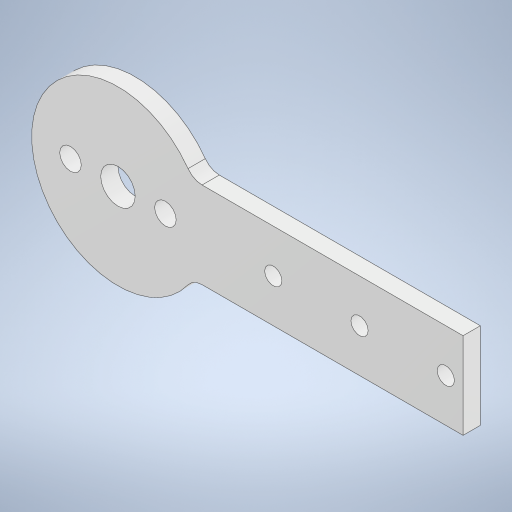
# Autodesk Inventor part: cutter_board
Saved by Autodesk Inventor 2024 (Build 280153000, 153)
## iProperties
Created: 2025-03-05
Part Number: cutter_board
Material: ABS プラスチック
Document SubType Name: Modeling
Designer: 1412z
Density: 1.06 g/cm^3
Appearance: 滑らか - 白
Author: 1412z
Autodesk Inventor part; units mm, degrees
ref_plane "YZ Plane" through (0, 0, 0) normal (1, 0, 0) x (0, 1, 0)
ref_plane "XZ Plane" through (0, 0, 0) normal (0, 1, 0) x (-1, 0, 0)
ref_plane "XY Plane" through (0, 0, 0) normal (0, 0, 1) x (1, 0, 0)
sketch "スケッチ5" plane through (0, 0, 0) normal (0, 0, 1) x (1, 0, 0)
  circle A0 centre (0, 0) radius 2
  circle A1 centre (0, 0) radius 10
  line L0 (0, 0) -> (40, 0)
  line L1 (40, 0) -> (40, -5)
  line L2 (40, -5) -> (8.6603, -5)
  line L3 (40, 0) -> (40, 5)
  line L4 (40, 5) -> (8.6603, 5)
  circle A2 centre (18, 0) radius 1
  circle A3 centre (28, 0) radius 1
  circle A4 centre (38, 0) radius 1
  circle A5 centre (0, 0) radius 5.5
  circle A6 centre (-5.5, 0) radius 1.25
  circle A7 centre (5.5, 0) radius 1.25
  dimension "d31" = 4
  dimension "d32" = 20
  dimension "d33" = 40
  dimension "d34" = 5
  dimension "d35" = 5
  dimension "d36" = 2
  dimension "d37" = 2
  dimension "d38" = 2
  dimension "d39" = 11
  dimension "d40" = 2.5
  dimension "d41" = 2.5
  constraints: 10 end point, 8 centre point, 5 point on line, 4 point on circle, 3 coincident, 3 perpendicular, 1 horizontal
  measures "d31" diameter of A0
  measures "d32" diameter of A1
  measures "d33" distance of L0.start L0.end
  measures "d34" distance of L0.end L1.end
  measures "d35" distance of L0.end L3.end
  measures "d36" diameter of A2
  measures "d37" diameter of A3
  measures "d38" diameter of A4
  measures "d39" diameter of A5
  measures "d40" diameter of A6
  measures "d41" diameter of A7
extrude "押し出し5" add sketch "スケッチ5" along normal blind 2 contours A7 A5 A6 | A1 | A1 L4 L3 L0 A4 A3 A2 | L0 A2 A3 A4 L1 L2 A1
fillet "フィレット2" radius 2 2 edges at (8.6603, 5, 1) (8.6603, -5, 1)
